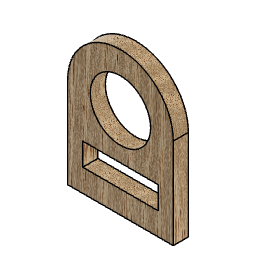
Ex1 (Autodesk Fusion 360 design; units mm, degrees)
Autodesk Fusion 360 part; units mm, degrees
sketch "Sketch1" plane through (0, 0, 0) normal (0, 1, 0) x (1, 0, 0) in component "Component'"
  circle A0 centre (0, 0) radius 20
  line L0 (0, 0) -> (0, 20)
  line L1 (-35, 0) -> (-35, 60)
  line L2 (-35, 60) -> (35, 60)
  line L3 (35, 60) -> (35, 0)
  arc A1 (-35, 0) -> (35, 0) centre (0, 0) ccw
  line L4 (0, 20) -> (0, 37.5) construction
  line L5 (25, 45) -> (-25, 45)
  line L6 (-25, 45) -> (-25, 30)
  line L7 (-25, 30) -> (25, 30)
  line L8 (25, 30) -> (25, 45)
  line L9 (25, 45) -> (-25, 30) construction
  line L10 (-25, 45) -> (25, 30) construction
  point P0 (0, 37.5)
  dimension "d1" = 40
  dimension "d2" = 70
  dimension "d4" = 70
  dimension "d5" = 17.5
  dimension "d6" = 50
  dimension "d7" = 15
  constraint coincident A0.centre L0.start
  constraint concentric A0 A1
  constraint vertical L0
  constraint tangent L1 A1
  constraint parallel L0 L1
  constraint perpendicular L0 L2
  constraint tangent L3 A1
  constraint perpendicular L2 L3
  constraint coincident A0 L0.end
  constraint parallel L0 L4
  constraint horizontal L5
  constraint perpendicular L5 L6
  constraint parallel L5 L7
  constraint parallel L6 L8
  constraint coincident L9 P0
  constraint coincident L10 P0
  constraint coincident P0 L4.end
  measures "d1" diameter of A0
  measures "d2" diameter of A1
  measures "d4" distance of L1.end L2.end
  measures "d5" distance of L0.end P0
  measures "d6" distance of L6.end L7.end
  measures "d7" distance of L5.end L6.end
sketch "Sketch2" plane through (0, 0, 0) normal (0, 1, 0) x (1, 0, 0) in component "Component'"
extrude "Extrude1" add sketch "Sketch1" along normal blind 10
component "Component" placed x (1, 0, 0) y (0, 1, 0) z (0, 0, 1) at (0, 0, 0)
component "Component'" placed x (1, 0, 0) y (0, 1, 0) z (0, 0, 1) at (0, 0, 0) in component "Component"
